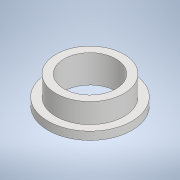
# Autodesk Inventor part: Упор
Saved by Autodesk Inventor 2021 (Build 250183000, 183)
## iProperties
Created: 2024-03-30
Part Number: Упор
Material: Типовые
Document SubType Name: Modeling
Designer: Мария
Density: 1 g/cm^3
Appearance: По умолчанию
Author: Мария
Autodesk Inventor part; units mm, degrees
ref_plane "YZ Plane" through (0, 0, 0) normal (1, 0, 0) x (0, 1, 0)
ref_plane "XZ Plane" through (0, 0, 0) normal (0, 1, 0) x (-1, 0, 0)
ref_plane "XY Plane" through (0, 0, 0) normal (0, 0, 1) x (1, 0, 0)
sketch "Эскиз1" plane through (0, 0, 0) normal (0, 0, 1) x (1, 0, 0)
  line L0 (6.5, 0) -> (6.5, 7)
  line L1 (6.5, 7) -> (8.5, 7)
  line L2 (8.5, 7) -> (8.5, 2)
  line L3 (8.5, 2) -> (10.5, 2)
  line L4 (10.5, 2) -> (10.5, 0)
  line L5 (10.5, 0) -> (6.5, 0)
  line L6 (0, 0) -> (0, 10)
  dimension "d0" = 10
  dimension "d1" = 13
  dimension "d2" = 4
  dimension "d4" = 2
  dimension "d7" = 2
  dimension "d8" = 5
  constraints: 14 end point, 4 perpendicular, 2 vertical, 1 horizontal alignment
  measures "d0" distance of L6.start L6.end
  measures "d1" diameter of L0 L6
  measures "d2" distance between parallel lines of L0 L4
  measures "d4" distance of L0.end L1.end
  measures "d7" distance of L3.end L4.end
  measures "d8" distance of L1.end L2.end
revolve "Вращение1" add sketch "Эскиз1" angle 360 about axis through (0, 0, 0) along (0, 1, 0)
